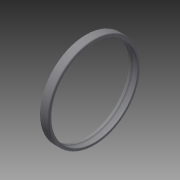
# Autodesk Inventor part: 61816_PART2
Saved by Autodesk Inventor 2014 SP2 (Build 180246200, 246)
## iProperties
Created: 2020-03-09
Part Number: 61816_PART2
Material: Generic
Catalog Web Link: www.cadenas.de
Description: -Deep groove ball bearings
Vendor: SKF
Document SubType Name: Modeling
Designer: psadmin
Manufacturer: SKF
Mass: 8.52437 g
Surface Area: 77.0675 cm^2
Volume: 8.52437 cm^3
Density: 1 g/cm^3
Appearance: PSOLRGB-175-175-175
Category: PARTsolutions
Company: SKF
Title: 61816_PART2
Author: Cadenas PARTsolutions
Comments: Deep groove ball bearings
PSOL_IDENT_0: {$CADENAS_DATA\23d-libs\skf\bearings_units_and_housings\ball_bearings\deep_groove_ball_bearings\bb1_
PSOL_IDENT_1: 001_101.prj},188 {VTYP=3D},{NB=61816_PART2},{LINA=61816_PART2},{NN=BB1_001_101_PART2},{NOPRJ=TRUE},{
PSOL_IDENT_2: DATE=19.12.2019 14:34:47},{GEOMDATE=18.12.2019 13:53:11},{VERSION=},{LINEID=6650},{WBVAR=},{WBNUMERI
PSOL_IDENT_3: C=}  {NB=61816_PART2},{LINA=61816_PART2},{KT=DUMMY},{PRODUCTID=1010021816},{DESIGNATION=61816},{DD=8
PSOL_IDENT_4: 0.000},{D=100.000},{B=10.000},{C=0.000},{DD1=86.70},{DD2=0.00},{D1=0.00},{D2=95.70},{D3=0.000},{D4=0
PSOL_IDENT_5: .000},{HH=MIN},{BB=0.000},{FF=0.00},{R0MAX=MIN},{R0=MIN},{R12=1.30},{PITCH=90.00},{DW=5.556},{DDAMIN=
PSOL_IDENT_6: 83.200},{DDAMAX=MIN},{DDBMIN=MIN},{DDBMAX=MIN},{DBMIN=MIN},{DAMAX=96.800},{BBAMIN=MIN},{CAMAX=MIN},{
PSOL_IDENT_7: RAMAX=0.600},{LOAD1=12.700},{LOAD2=11.200},{LOAD3=0.610},{SPEED1=13000},{SPEED2=8000},{KR=0.015},{F0=
PSOL_IDENT_8: 13.300},{Z=27},{II=1},{MASS=0.153},{BEARING=61816},{RING=},{HELP=3.139},{HELP2=2.150},{DD1ALG=43.350
PSOL_IDENT_9: },{YALG=43.350},{PITCH1=90.000},{DW1=5.556},{YALG1=46.861},{HALG1=3.139},{SH=43.350},{CU=0.889},{DES
PSOL_IDENT_10: IGN=dgbb1},{HALG=3.35},{B1=0},{SHIELDHELP=1}
NT: Deep groove ball bearings
NB: 61816_PART2
NBSYN: $DESIGNATION._PART2
LINA: 61816_PART2
SUPPLIER: SKF
ARTICLENO: 61816_PART2
BOMINFO: 61816_PART2
CREATOR: CADENAS GmbH
Autodesk Inventor part; units mm, degrees
ref_plane "YZ Plane" through (0, 0, 0) normal (1, 0, 0) x (0, 1, 0)
ref_plane "XZ Plane" through (0, 0, 0) normal (0, 1, 0) x (-1, 0, 0)
ref_plane "XY Plane" through (0, 0, 0) normal (0, 0, 1) x (1, 0, 0)
sketch "Sketch_1" plane through (0, 0, 0) normal (0, 0, 1) x (1, 0, 0)
  line L0 (50, 0) -> (-50, 0)
  line L1 (0, 48.7) -> (0, 47.2943)
  arc A0 (0, 47.2943) -> (0.4333, 46.861) centre (0.4333, 47.2943) ccw
  line L2 (0.4333, 46.861) -> (2.9375, 46.861)
  arc A1 (7.0625, 46.861) -> (2.9375, 46.861) centre (5, 45) ccw
  line L3 (7.0625, 46.861) -> (9.5667, 46.861)
  arc A2 (9.5667, 46.861) -> (10, 47.2943) centre (9.5667, 47.2943) ccw
  line L4 (10, 47.2943) -> (10, 48.7)
  arc A3 (10, 48.7) -> (8.7, 50) centre (8.7, 48.7) ccw
  line L5 (8.7, 50) -> (1.3, 50)
  arc A4 (1.3, 50) -> (0, 48.7) centre (1.3, 48.7) ccw
  constraints: 12 end point, 10 point on circle, 5 centre point
revolve "Revolution1" add sketch "Sketch_1" angle 360 about axis through (50, 0, 0) along (1, 0, 0)
body "Solid1"
